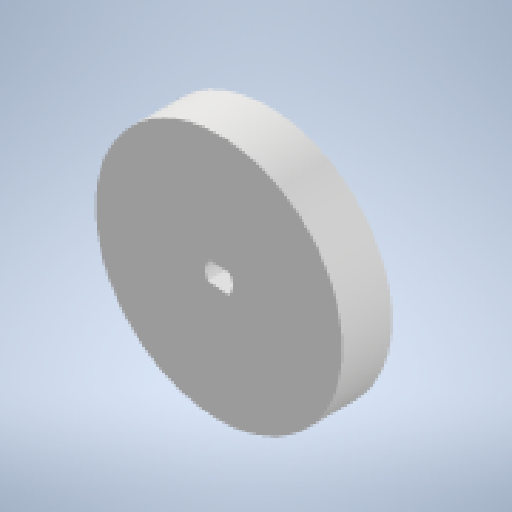
# Autodesk Inventor part: Wheel
Saved by Autodesk Inventor 2024 (Build 280153000, 153)
## iProperties
Created: 2025-06-20
Part Number: Wheel
Material: Generic
Document SubType Name: Modeling
Designer: Aidan
Density: 1 g/cm^3
Appearance: Default
Author: Aidan
Autodesk Inventor part; units mm, degrees
ref_plane "YZ Plane" through (0, 0, 0) normal (1, 0, 0) x (0, 1, 0)
ref_plane "XZ Plane" through (0, 0, 0) normal (0, 1, 0) x (-1, 0, 0)
ref_plane "XY Plane" through (0, 0, 0) normal (0, 0, 1) x (1, 0, 0)
sketch "Sketch1" plane through (0, 0, 0) normal (0, 0, 1) x (1, 0, 0)
  arc A0 (3.5439, 9.7114) -> (3.9233, 13.2109) centre (1.7309, 11.6783) ccw projected
  line L0 (3.9233, 13.2109) -> (-0.0821, 13.6452) projected
  arc A1 (-0.0821, 13.6452) -> (-0.4616, 10.1457) centre (1.7309, 11.6783) ccw projected
  line L1 (-0.4616, 10.1457) -> (3.5439, 9.7114) projected
  circle A2 centre (1.7309, 11.6783) radius 1.04 projected
  circle A3 centre (1.7309, 11.6783) radius 25
  line L2 (-0.1489, 13.8536) -> (4.0332, 13.4001)
  arc A4 (3.6107, 9.503) -> (4.0332, 13.4001) centre (1.7309, 11.6783) ccw
  line L3 (3.6107, 9.503) -> (-0.5715, 9.9564)
  arc A5 (-0.1489, 13.8536) -> (-0.5715, 9.9564) centre (1.7309, 11.6783) ccw
  point P0 (0, 0)
  dimension "d0" = 50
  dimension "d1" = 0.2
  constraints: 4 end point, 4 point on circle, 3 centre point, 1 coincident, 3 other
  measures "d0" diameter of A3
  measures "d1" distance between parallel lines of L0 L2
extrude "Extrusion1" add sketch "Sketch1" along normal blind 15 contours A3
sketch "Sketch2" plane through (1.7309, 11.6783, 0) normal (0, 0, -1) x (-1, 0, 0)
  arc A0 (-2.3024, 1.7218) -> (-1.8798, -2.1753) centre (0, 0) ccw projected
  circle A1 centre (0, 0) radius 25 projected
  line L0 (-1.8798, -2.1753) -> (2.3024, -1.7218) projected
  arc A2 (-2.3024, 1.7218) -> (-1.8798, -2.1753) centre (0, 0) ccw projected
  line L1 (1.8798, 2.1753) -> (-2.3024, 1.7218) projected
  arc A3 (2.3024, -1.7218) -> (1.8798, 2.1753) centre (0, 0) ccw projected
  circle A4 centre (0, 0) radius 5
  circle A5 centre (0, 0) radius 25
  point P0 (1.7309, -11.6783)
  dimension "d4" = 10
  constraints: 2 centre point, 2 coincident, 1 concentric
  measures "d4" diameter of A4
extrude "Extrusion2" cut sketch "Sketch2" against normal blind 7.5 contours A1
body "Solid1"
